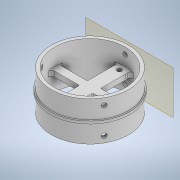
# Autodesk Inventor part: Verbindungsring_2_3
Saved by Autodesk Inventor 2020 (Build 240168000, 168)
## iProperties
Created: 2022-02-05
Part Number: Verbindungsring_2_3
Material: Generisch
Document SubType Name: Modeling
Designer: sp
Density: 1 g/cm^3
Appearance: Vorgabe
Author: sp
Autodesk Inventor part; units mm, degrees
ref_plane "YZ Plane" through (0, 0, 0) normal (1, 0, 0) x (0, 1, 0)
ref_plane "XZ Plane" through (0, 0, 0) normal (0, 1, 0) x (-1, 0, 0)
sketch "Skizze5" plane through (0, 0, 0) normal (0, 1, 0) x (-1, 0, 0)
  circle A0 centre (0, 0) radius 27
  circle A1 centre (0, 0) radius 30.5
  dimension "d23" = 61
  dimension "d24" = 54
  constraints: 2 centre point, 2 coincident
  measures "d23" diameter of A1
  measures "d24" diameter of A0
extrude "Extrusion4" add sketch "Skizze5" along normal mid plane 2
sketch "Skizze6" plane through (0, 0, 0) normal (0, 1, 0) x (-1, 0, 0)
  circle A0 centre (0, 0) radius 27
  circle A1 centre (0, 0) radius 29.5
  dimension "d27" = 54
  dimension "d28" = 59
  constraints: 2 centre point, 2 coincident
  measures "d27" diameter of A0
  measures "d28" diameter of A1
extrude "Extrusion5" add sketch "Skizze6" along normal mid plane 30
ref_plane "Arbeitsebene5" through (0, 0, -30) normal (0, 0, 1) x (1, 0, 0)
sketch "Skizze7" plane through (0, 0, -30) normal (0, 0, 1) x (1, 0, 0)
  circle A0 centre (0, -10) radius 1.75
  circle A1 centre (0, 10) radius 1.75
  line L0 (-34.5015, 0) -> (40.4508, 0) construction
  point P0 (0, 0)
  dimension "d32" = 3.5
  dimension "d33" = 3.5
  dimension "d34" = 20
  constraints: 2 centre point, 2 end point, 1 horizontal, 1 point on line, 1 symmetric about line
  measures "d32" diameter of A0
  measures "d33" diameter of A1
  measures "d34" distance of A1.centre A0.centre
extrude "Extrusion6" cut sketch "Skizze7" along normal blind 5
pattern_circular "Runde Anordnung2" count 3 over 360 about axis through (0, -10, 0) along (0, 1, 0) of "Extrusion6"
sketch "Skizze8" plane through (0, 0, 0) normal (0, 1, 0) x (-1, 0, 0)
  line L0 (-16.7844, 0) -> (18.1163, 0) construction
  line L1 (0, -12.3348) -> (0, 12.3348) construction
  circle A0 centre (0, -22.5) radius 1.75
  circle A1 centre (0, 22.5) radius 1.75
  circle A2 centre (0, -22.5) radius 5
  circle A3 centre (0, 22.5) radius 5
  line L2 (-5, -22.5) -> (5, -22.5)
  line L3 (5, -22.5) -> (5, 22.5)
  line L4 (5, 22.5) -> (-5, 22.5)
  line L5 (-5, 22.5) -> (-5, -22.5)
  circle A4 centre (0, 0) radius 27.0734
  line L6 (-29, -3) -> (29, -3)
  line L7 (29, -3) -> (29, 3)
  line L8 (29, 3) -> (-29, 3)
  line L9 (-29, 3) -> (-29, -3)
  point P0 (5, -3)
  point P1 (26.9066, -3)
  point P2 (26.9066, 3)
  point P3 (5, 3)
  point P4 (2.215, 26.9826)
  point P5 (-2.215, 26.9826)
  point P6 (-5, 3)
  point P7 (-26.9066, 3)
  point P8 (-26.9066, -3)
  point P9 (-5, -3)
  point P10 (-2.215, -26.9826)
  point P11 (2.215, -26.9826)
  dimension "d43" = 10
  dimension "d44" = 10
  dimension "d40" = 3.5
  dimension "d41" = 3.5
  dimension "d42" = 45
  dimension "d45" = 6
  dimension "d46" = 58
  constraints: 20 end point, 4 parallel, 3 centre point, 3 coincident, 3 horizontal, 3 point on line, 2 perpendicular, 1 midpoint, 1 symmetric about line, 1 vertical, 8 other
  measures "d40" diameter of A0
  measures "d41" diameter of A1
  measures "d42" distance of A1.centre A0.centre
  measures "d45" distance of L6.end L7.end
  measures "d46" distance of L7.end L8.end
extrude "Extrusion7" add sketch "Skizze8" along normal mid plane 4 contours L2 A2 A4 A0 | A0 L2 A2 | A2 L5 L6 L3 | L6 L5 L8 L3 | L3 L8 A4 L6 | L6 A4 L8 L5 | L8 L5 A3 L3 | L4 A1 A3 A4 | A3 L4 A1
fillet "Rundung2" radius 2 16 edges at (2.3851, 1.5, 26.8944) (2.3851, -1.5, 26.8944) (2.3851, 0.5, 26.8944) (2.3851, -0.5, 26.8944) (-2.3851, 1.5, 26.8944) (-2.3851, -1.5, 26.8944) (-2.3851, 0.5, 26.8944) (-2.3851, -0.5, 26.8944) (-2.3851, 1.5, -26.8944) (-2.3851, -1.5, -26.8944) (-2.3851, 0.5, -26.8944) (-2.3851, -0.5, -26.8944) (2.3851, 1.5, -26.8944) (2.3851, -1.5, -26.8944) (2.3851, 0.5, -26.8944) (2.3851, -0.5, -26.8944)
fillet "Rundung3" radius 2 16 edges at (26.8328, 1.5, -3) (26.8328, 0.5, -3) (26.8328, -0.5, -3) (26.8328, -1.5, -3) (26.8328, 1.5, 3) (26.8328, 0.5, 3) (26.8328, -1.5, 3) (26.8328, -0.5, 3) (-26.8328, 1.5, -3) (-26.8328, -1.5, -3) (-26.8328, -0.5, -3) (-26.8328, 0.5, -3) (-26.8328, 1.5, 3) (-26.8328, 0.5, 3) (-26.8328, -0.5, 3) (-26.8328, -1.5, 3)
fillet "Rundung4" radius 1 4 edges at (5, 0, -3) (5, 0, 3) (-5, 0, 3) (-5, 0, -3)
